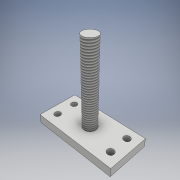
# Autodesk Inventor part: Male for pack
Saved by Autodesk Inventor 2018.1 (Build 221171000, 171)
## iProperties
Created: 2019-01-30
Part Number: Male for pack
Material: Типовые
Document SubType Name: Modeling
Designer: kostya
Density: 1 g/cm^3
Appearance: По умолчанию
Author: kostya
Autodesk Inventor part; units mm, degrees
ref_plane "YZ Plane" through (0, 0, 0) normal (1, 0, 0) x (0, 1, 0)
ref_plane "XZ Plane" through (0, 0, 0) normal (0, 1, 0) x (-1, 0, 0)
ref_plane "XY Plane" through (0, 0, 0) normal (0, 0, 1) x (1, 0, 0)
sketch "Эскиз1" plane through (0, 0, 0) normal (0, 0, 1) x (1, 0, 0)
  circle A0 centre (0, 0) radius 3
  dimension "d0" = 6
  constraints: 1 centre point, 1 coincident
  measures "d0" diameter of A0
extrude "Выдавливание1" add sketch "Эскиз1" along normal blind 36
sketch "Эскиз2" plane through (0, 0, 0) normal (0, 0, -1) x (-1, 0, 0)
  line L0 (-18, -9) -> (18, -9)
  line L1 (18, -9) -> (18, 9)
  line L2 (18, 9) -> (-18, 9)
  line L3 (-18, 9) -> (-18, -9)
  line L4 (-18, -9) -> (18, 9) construction
  line L5 (18, -9) -> (-18, 9) construction
  line L6 (0, 9) -> (0, 0) construction
  line L7 (0, 0) -> (0, -9) construction
  line L8 (0, 4.5) -> (-15, 4.5) construction
  line L9 (-15, 4.5) -> (-12, 4.5) construction
  circle A0 centre (-13.5, 4.5) radius 1.5
  line L10 (-13.5, 6) -> (-13.5, -5.5) construction
  line L11 (-13.5, -5.5) -> (-13.5, -2.5) construction
  circle A1 centre (-13.5, -4) radius 1.5
  circle A2 centre (13.5, 4.5) radius 1.5
  line L12 (13.5, 6) -> (13.5, -5.5) construction
  line L13 (13.5, -5.5) -> (13.5, -2.5) construction
  circle A3 centre (13.5, -4) radius 1.5
  dimension "d3" = 36
  dimension "d4" = 18
  dimension "d5" = 15
  dimension "d6" = 3
  dimension "d7" = 11.5
  dimension "d8" = 3
  constraints: 28 end point, 7 midpoint, 5 symmetric about line, 3 vertical, 3 vertical alignment, 2 horizontal, 2 parallel, 2 point on circle, 2 point on line, 1 centre point, 1 perpendicular, 7 other
  measures "d3" distance of L2.end L1.end
  measures "d4" distance of L1.end L0.end
  measures "d5" distance of L8.start L8.end
  measures "d6" distance of L8.end L9.end
  measures "d7" distance of L10.start L10.end
  measures "d8" distance of L10.end L11.end
extrude "Выдавливание2" add sketch "Эскиз2" along normal blind 4
thread "Резьба1" size "M6x1" class "6g" standard "ANSI Metric M Profile" full length
